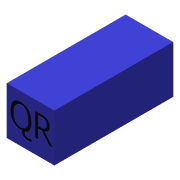
# Autodesk Inventor part: Container 1 1 2 and half
Saved by Autodesk Inventor 2015 (Build 190159000, 159)
## iProperties
Created: 2015-03-07
Part Number: Container 1 1 2 and half
Material: Generic
Document SubType Name: Modeling
Designer: Vukica
Density: 1 g/cm^3
Appearance: Default
Author: Vukica
Autodesk Inventor part; units mm, degrees
ref_plane "YZ Plane" through (0, 0, 0) normal (1, 0, 0) x (0, 1, 0)
ref_plane "XZ Plane" through (0, 0, 0) normal (0, 1, 0) x (-1, 0, 0)
ref_plane "XY Plane" through (0, 0, 0) normal (0, 0, 1) x (1, 0, 0)
sketch "Sketch1" plane through (0, 0, 0) normal (0, 0, 1) x (1, 0, 0)
  line L0 (0, 0) -> (25.4, 0)
  line L1 (25.4, 0) -> (25.4, 25.4)
  line L2 (25.4, 25.4) -> (0, 25.4)
  line L3 (0, 25.4) -> (0, 0)
  dimension "d0" = 25.4
  dimension "d1" = 25.4
  constraints: 8 end point, 2 parallel, 1 horizontal, 1 perpendicular
  measures "d0" distance of L1.end L2.end
  measures "d1" distance of L2.end L0.start
extrude "Extrusion1" add sketch "Sketch1" along normal blind 63.5
sketch "Sketch2" plane through (0, 0, 63.5) normal (0, 0, 1) x (1, 0, 0)
  line L0 (1.2774, 20.3944) -> (24.475, 20.3944) construction
  line L1 (24.475, 20.3944) -> (24.475, 4.082) construction
  line L2 (24.475, 4.082) -> (1.2774, 4.082) construction
  line L3 (1.2774, 4.082) -> (1.2774, 20.3944) construction
  spline S0 degree 2 poles (13.1129, 4.3187) (12.6498, 4.2055) (11.6412, 4.082) (11.1369, 4.082) knots 0 0 0 1 2 2 2
  spline S1 degree 2 poles (11.1369, 4.082) (9.7063, 4.082) (7.9259, 5.6772) (7.8435, 7.1592) knots 0 0 0 1 2 2 2
  spline S2 degree 2 poles (7.8435, 7.1592) (7.7303, 7.1592) (7.5348, 7.1592) (7.4524, 7.1592) knots 0 0 0 1 2 2 2
  spline S3 degree 2 poles (7.4524, 7.1592) (6.166, 7.1592) (4.0973, 8.034) (3.3563, 8.8882) knots 0 0 0 1 2 2 2
  spline S4 degree 2 poles (3.3563, 8.8882) (2.6256, 9.7321) (1.8434, 12.2022) (1.8434, 13.7665) knots 0 0 0 1 2 2 2
  spline S5 degree 2 poles (1.8434, 13.7665) (1.8434, 15.372) (2.6359, 17.8009) (3.3666, 18.6654) knots 0 0 0 1 2 2 2
  spline S6 degree 2 poles (3.3666, 18.6654) (4.1076, 19.5196) (6.1763, 20.3944) (7.4524, 20.3944) knots 0 0 0 1 2 2 2
  spline S7 degree 2 poles (7.4524, 20.3944) (8.7492, 20.3944) (10.8281, 19.4887) (11.5486, 18.6654) knots 0 0 0 1 2 2 2
  spline S8 degree 2 poles (11.5486, 18.6654) (12.269, 17.8317) (13.0717, 15.3514) (13.0717, 13.7665) knots 0 0 0 1 2 2 2
  spline S9 degree 2 poles (13.0717, 13.7665) (13.0717, 11.2965) (11.1472, 8.0855) (9.4696, 7.5194) knots 0 0 0 1 2 2 2
  spline S10 degree 2 poles (9.4696, 7.5194) (9.5108, 7.046) (9.7578, 6.2844) (9.9533, 6.0683) knots 0 0 0 1 2 2 2
  spline S11 degree 2 poles (9.9533, 6.0683) (10.19, 5.8007) (10.8384, 5.5537) (11.4148, 5.5537) knots 0 0 0 1 2 2 2
  spline S12 degree 2 poles (11.4148, 5.5537) (11.7544, 5.5537) (12.6806, 5.7698) (12.8865, 5.8522) knots 0 0 0 1 2 2 2
  line L4 (12.8865, 5.8522) -> (13.1129, 5.8522)
  line L5 (13.1129, 5.8522) -> (13.1129, 4.3187)
  spline S13 degree 2 poles (11.3118, 13.7665) (11.3118, 15.0324) (10.7664, 16.9775) (10.2724, 17.6156) knots 0 0 0 1 2 2 2
  spline S14 degree 2 poles (10.2724, 17.6156) (9.7681, 18.2743) (8.3478, 18.933) (7.4627, 18.933) knots 0 0 0 1 2 2 2
  spline S15 degree 2 poles (7.4627, 18.933) (6.5468, 18.933) (5.1677, 18.2949) (4.6428, 17.6156) knots 0 0 0 1 2 2 2
  spline S16 degree 2 poles (4.6428, 17.6156) (4.1385, 16.9672) (3.6033, 15.0015) (3.6033, 13.7665) knots 0 0 0 1 2 2 2
  spline S17 degree 2 poles (3.6033, 13.7665) (3.6033, 11.2656) (5.7028, 8.6001) (7.4627, 8.6001) knots 0 0 0 1 2 2 2
  spline S18 degree 2 poles (7.4627, 8.6001) (9.2226, 8.6001) (11.3118, 11.2656) (11.3118, 13.7665) knots 0 0 0 1 2 2 2
  line L6 (24.7528, 7.4268) -> (22.5607, 7.4268)
  line L7 (22.5607, 7.4268) -> (18.5469, 12.48)
  line L8 (18.5469, 12.48) -> (16.6121, 12.48)
  line L9 (16.6121, 12.48) -> (16.6121, 7.4268)
  line L10 (16.6121, 7.4268) -> (14.9242, 7.4268)
  line L11 (14.9242, 7.4268) -> (14.9242, 20.1268)
  line L12 (14.9242, 20.1268) -> (18.197, 20.1268)
  spline S19 degree 2 poles (18.197, 20.1268) (19.2879, 20.1268) (20.7597, 19.8901) (21.4286, 19.4578) knots 0 0 0 1 2 2 2
  spline S20 degree 2 poles (21.4286, 19.4578) (22.0976, 19.0256) (22.8695, 17.6774) (22.8695, 16.6791) knots 0 0 0 1 2 2 2
  spline S21 degree 2 poles (22.8695, 16.6791) (22.8695, 15.2897) (21.4492, 13.4063) (20.2348, 12.9535) knots 0 0 0 1 2 2 2
  line L13 (20.2348, 12.9535) -> (24.7528, 7.4268)
  spline S22 degree 2 poles (21.1096, 16.5453) (21.1096, 17.101) (20.7185, 17.9552) (20.3068, 18.2331) knots 0 0 0 1 2 2 2
  spline S23 degree 2 poles (20.3068, 18.2331) (19.9466, 18.4698) (18.9895, 18.6654) (18.2896, 18.6654) knots 0 0 0 1 2 2 2
  line L14 (18.2896, 18.6654) -> (16.6121, 18.6654)
  line L15 (16.6121, 18.6654) -> (16.6121, 13.89)
  line L16 (16.6121, 13.89) -> (18.0941, 13.89)
  spline S24 degree 2 poles (18.0941, 13.89) (18.8248, 13.89) (19.9878, 14.1473) (20.3892, 14.5487) knots 0 0 0 1 2 2 2
  spline S25 degree 2 poles (20.3892, 14.5487) (20.7597, 14.8986) (21.1096, 15.8866) (21.1096, 16.5453) knots 0 0 0 1 2 2 2
  point P0 (0, 0)
  constraints: 2 other
extrude "Extrusion2" cut sketch "Sketch2" against normal blind 0.254
equation "\"d1\" = d0"
body "Solid1"
